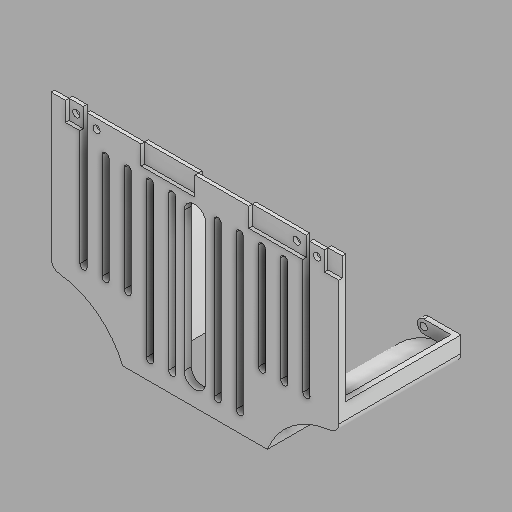
# Autodesk Inventor part: RC_CAR_TOP_PLATE
Saved by Autodesk Inventor 2025.2 (Build 292293000, 293)
## iProperties
Created: 2025-10-26
Part Number: RC_CAR_TOP_PLATE
Material: Generic
Document SubType Name: Modeling
Designer: Ben
Density: 1 g/cm^3
Appearance: Default
Author: Ben
Autodesk Inventor part; units mm, degrees
ref_plane "YZ Plane" through (0, 0, 0) normal (1, 0, 0) x (0, 1, 0)
ref_plane "XZ Plane" through (0, 0, 0) normal (0, 1, 0) x (-1, 0, 0)
ref_plane "XY Plane" through (0, 0, 0) normal (0, 0, 1) x (1, 0, 0)
sketch "Sketch1" plane through (0, 0, 0) normal (0, 0, 1) x (1, 0, 0)
  line L0 (-133.35, 0) -> (133.35, 0) projected
  line L1 (0, -231.14) -> (0, 231.14) projected
  line L2 (-44.45, -165.1) -> (44.45, 165.1) construction
  line L3 (44.45, -165.1) -> (-44.45, 165.1) construction
  line L4 (-95.25, -88.9) -> (-44.45, -88.9)
  line L5 (-44.45, 88.9) -> (-95.25, 88.9)
  line L6 (-95.25, 88.9) -> (-95.25, -88.9)
  line L7 (-95.25, -88.9) -> (-44.45, 88.9) construction
  line L8 (-44.45, -88.9) -> (-95.25, 88.9) construction
  line L9 (95.25, -88.9) -> (44.45, -88.9)
  line L10 (44.45, 88.9) -> (95.25, 88.9)
  line L11 (95.25, 88.9) -> (95.25, -88.9)
  line L12 (95.25, -88.9) -> (44.45, 88.9) construction
  line L13 (44.45, -88.9) -> (95.25, 88.9) construction
  line L14 (44.45, -165.1) -> (44.45, -88.9)
  line L15 (44.45, 88.9) -> (44.45, 165.1)
  line L16 (-44.45, 165.1) -> (-44.45, 88.9)
  line L17 (-44.45, -88.9) -> (-44.45, -165.1)
  line L18 (-31.75, 120.65) -> (31.75, 120.65)
  line L19 (31.75, 120.65) -> (31.75, 165.1)
  line L20 (-31.75, 165.1) -> (-31.75, 120.65)
  line L21 (-31.75, 120.65) -> (31.75, 165.1) construction
  line L22 (31.75, 120.65) -> (-31.75, 165.1) construction
  line L23 (-31.75, -120.65) -> (31.75, -120.65)
  line L24 (31.75, -120.65) -> (31.75, -165.1)
  line L25 (-31.75, -165.1) -> (-31.75, -120.65)
  line L26 (-31.75, -120.65) -> (31.75, -165.1) construction
  line L27 (31.75, -120.65) -> (-31.75, -165.1) construction
  line L28 (44.45, 165.1) -> (31.75, 165.1)
  line L29 (-31.75, 165.1) -> (-44.45, 165.1)
  line L30 (-44.45, -165.1) -> (-31.75, -165.1)
  line L31 (31.75, -165.1) -> (44.45, -165.1)
  point P0 (0, 0)
  point P1 (-69.85, 0)
  point P2 (69.85, 0)
  point P3 (0, 142.875)
  point P4 (0, -142.875)
  dimension "d0" = 88.9
  dimension "d1" = 330.2
  dimension "d3" = 50.8
  dimension "d4" = 12.7
  dimension "d5" = 44.45
  dimension "d27" = 76.2
  constraints: 60 end point, 12 parallel, 10 midpoint, 6 horizontal, 6 perpendicular, 4 point on line, 4 other
  measures "d0" distance of L2.end L3.end
  measures "d1" distance of L3.end L2.start
  measures "d3" distance of L4.start L4.end
  measures "d4" distance between parallel lines of L16 L20
  measures "d5" distance of L20.start L18.start
  measures "d27" distance between parallel lines of L29 L5
extrude "Extrusion1" add sketch "Sketch1" along normal blind 4.7625
sketch "Sketch3" plane through (0, 0, 4.7625) normal (0, 0, 1) x (1, 0, 0)
  line L0 (73.8188, -76.2) -> (73.8187, 76.2) construction
  line L1 (76.2, -76.2) -> (76.2, 76.2)
  line L2 (71.4375, 76.2) -> (71.4375, -76.2)
  arc A0 (71.4375, -76.2) -> (76.2, -76.2) centre (73.8188, -76.2) ccw
  arc A1 (76.2, 76.2) -> (71.4375, 76.2) centre (73.8187, 76.2) ccw
  line L3 (-73.8188, -76.2) -> (-73.8188, 76.2) construction
  line L4 (-71.4375, -76.2) -> (-71.4375, 76.2)
  line L5 (-76.2, 76.2) -> (-76.2, -76.2)
  arc A2 (-76.2, -76.2) -> (-71.4375, -76.2) centre (-73.8188, -76.2) ccw
  arc A3 (-71.4375, 76.2) -> (-76.2, 76.2) centre (-73.8188, 76.2) ccw
  line L6 (0, -231.14) -> (0, 231.14) projected
  line L7 (-133.35, 0) -> (133.35, 0) projected
  line L8 (95.25, -88.9) -> (95.25, 88.9) projected
  line L9 (59.1344, -76.2) -> (59.1344, -6.35) construction
  line L10 (61.5156, -76.2) -> (61.5156, -6.35)
  line L11 (56.7531, -6.35) -> (56.7531, -76.2)
  arc A4 (56.7531, -76.2) -> (61.5156, -76.2) centre (59.1344, -76.2) ccw
  arc A5 (61.5156, -6.35) -> (56.7531, -6.35) centre (59.1344, -6.35) ccw
  line L12 (44.45, -76.2) -> (44.45, -6.35) construction
  line L13 (44.45, -165.1) -> (44.45, -88.9) projected
  line L14 (46.8313, -76.2) -> (46.8313, -6.35)
  line L15 (42.0688, -6.35) -> (42.0688, -76.2)
  arc A6 (42.0688, -76.2) -> (46.8313, -76.2) centre (44.45, -76.2) ccw
  arc A7 (46.8313, -6.35) -> (42.0688, -6.35) centre (44.45, -6.35) ccw
  line L16 (-59.1344, -76.2) -> (-59.1344, -6.35) construction
  line L17 (-56.7531, -76.2) -> (-56.7531, -6.35)
  line L18 (-61.5156, -6.35) -> (-61.5156, -76.2)
  arc A8 (-61.5156, -76.2) -> (-56.7531, -76.2) centre (-59.1344, -76.2) ccw
  arc A9 (-56.7531, -6.35) -> (-61.5156, -6.35) centre (-59.1344, -6.35) ccw
  line L19 (-44.45, -76.2) -> (-44.45, -6.35) construction
  line L20 (-95.25, -88.9) -> (-44.45, -88.9) projected
  line L21 (-42.0687, -76.2) -> (-42.0687, -6.35)
  line L22 (-46.8313, -6.35) -> (-46.8313, -76.2)
  arc A10 (-46.8313, -76.2) -> (-42.0687, -76.2) centre (-44.45, -76.2) ccw
  arc A11 (-42.0687, -6.35) -> (-46.8313, -6.35) centre (-44.45, -6.35) ccw
  line L23 (-73.8188, -76.2) -> (-59.1344, -76.2) construction
  line L24 (-44.45, -76.2) -> (-59.1344, -76.2) construction
  line L25 (59.1344, -76.2) -> (44.45, -76.2) construction
  line L26 (73.8188, -76.2) -> (59.1344, -76.2) construction
  line L27 (29.7656, -107.95) -> (29.7656, -6.35) construction
  line L28 (44.45, 88.9) -> (44.45, 165.1) projected
  line L29 (32.1469, -107.95) -> (32.1469, -6.35)
  line L30 (27.3844, -6.35) -> (27.3844, -107.95)
  arc A12 (27.3844, -107.95) -> (32.1469, -107.95) centre (29.7656, -107.95) ccw
  arc A13 (32.1469, -6.35) -> (27.3844, -6.35) centre (29.7656, -6.35) ccw
  line L31 (-31.75, -120.65) -> (31.75, -120.65) projected
  line L32 (44.45, -76.2) -> (29.7656, -76.2) construction
  line L33 (-29.7656, -107.95) -> (-29.7656, -6.35) construction
  line L34 (-27.3844, -107.95) -> (-27.3844, -6.35)
  line L35 (-32.1469, -6.35) -> (-32.1469, -107.95)
  arc A14 (-32.1469, -107.95) -> (-27.3844, -107.95) centre (-29.7656, -107.95) ccw
  arc A15 (-27.3844, -6.35) -> (-32.1469, -6.35) centre (-29.7656, -6.35) ccw
  line L36 (-44.45, -76.2) -> (-29.7656, -76.2) construction
  line L37 (-15.0812, -107.95) -> (-15.0812, -6.35) construction
  line L38 (-12.7, -107.95) -> (-12.7, -6.35)
  line L39 (-17.4625, -6.35) -> (-17.4625, -107.95)
  arc A16 (-17.4625, -107.95) -> (-12.7, -107.95) centre (-15.0812, -107.95) ccw
  arc A17 (-12.7, -6.35) -> (-17.4625, -6.35) centre (-15.0812, -6.35) ccw
  line L40 (-29.7656, -76.2) -> (-15.0812, -76.2) construction
  line L41 (15.0812, -107.95) -> (15.0813, -6.35) construction
  line L42 (17.4625, -107.95) -> (17.4625, -6.35)
  line L43 (12.7, -6.35) -> (12.7, -107.95)
  arc A18 (12.7, -107.95) -> (17.4625, -107.95) centre (15.0812, -107.95) ccw
  arc A19 (17.4625, -6.35) -> (12.7, -6.35) centre (15.0813, -6.35) ccw
  line L44 (29.7656, -76.2) -> (15.0812, -76.2) construction
  line L45 (0, -103.1875) -> (0, -11.1125) construction
  line L46 (7.1438, -103.1875) -> (7.1438, -11.1125)
  line L47 (-7.1438, -11.1125) -> (-7.1438, -103.1875)
  arc A20 (-7.1438, -103.1875) -> (7.1438, -103.1875) centre (0, -103.1875) ccw
  arc A21 (7.1438, -11.1125) -> (-7.1438, -11.1125) centre (0, -11.1125) ccw
  line L48 (-29.7656, -110.3313) -> (29.7656, -110.3313) construction
  point P0 (0, 0)
  point P1 (73.8187, 0)
  point P2 (-73.8187, 0)
  point P3 (59.1344, -41.275)
  point P4 (44.45, -41.275)
  point P5 (-59.1344, -41.275)
  point P6 (-44.45, -41.275)
  point P7 (29.7656, -57.15)
  point P8 (-29.7656, -57.15)
  point P9 (-15.0812, -57.15)
  point P10 (15.0813, -57.15)
  point P11 (0, -57.15)
  point P12 (0, -110.3313)
  point P13 (-59.1344, -3.9687)
  point P14 (-44.45, -3.9687)
  point P15 (-29.7656, -3.9687)
  point P16 (-15.0812, -3.9687)
  point P17 (0, -3.9687)
  point P18 (15.0813, -3.9688)
  point P19 (29.7656, -3.9687)
  point P20 (44.45, -3.9688)
  point P21 (59.1344, -3.9688)
  dimension "d22" = 152.4
  dimension "d23" = 4.7625
  dimension "d24" = 19.05
  dimension "d51" = 12.7
  dimension "d53" = 14.2875
  dimension "d54" = 6.35
  constraints: 106 end point, 56 point on circle, 45 tangent, 22 centre point, 16 horizontal alignment, 14 parallel, 11 midpoint, 9 collinear, 8 equal radius, 8 perpendicular, 6 point on line, 4 vertical, 2 vertical alignment, 2 other
  measures "d22" distance of L0.end L0.start
  measures "d23" distance between parallel lines of L1 L2
  measures "d24" distance between parallel lines of L8 L1
  measures "d51" distance from line of L31 L27.start
  measures "d53" distance between parallel lines of L46 L47
  measures "d54" distance from line of L7 L12.end
extrude "Extrusion2" cut sketch "Sketch3" along normal through all both and the other way through all
fillet "Fillet1" radius 6.35 16 edges at (44.45, 165.1, 2.3813) (31.75, 165.1, 2.3813) (95.25, 88.9, 2.3813) (31.75, 120.65, 2.3813) (-31.75, 120.65, 2.3813) (-31.75, 165.1, 2.3813) (-44.45, 165.1, 2.3813) (-95.25, 88.9, 2.3813) (-95.25, -88.9, 2.3813) (-44.45, -165.1, 2.3813) (-31.75, -165.1, 2.3813) (-31.75, -120.65, 2.3813) (31.75, -120.65, 2.3813) (31.75, -165.1, 2.3813) (44.45, -165.1, 2.3813) (95.25, -88.9, 2.3813)
fillet "Fillet2" radius 50.8 4 edges at (44.45, -88.9, 2.3813) (-44.45, -88.9, 2.3813) (-44.45, 88.9, 2.3813) (44.45, 88.9, 2.3813)
sketch "Sketch4" plane through (0, 0, 4.7625) normal (0, 0, 1) x (1, 0, 0)
  line L0 (-133.35, 0) -> (133.35, 0) projected
  line L1 (0, -231.14) -> (0, 231.14) projected
  line L2 (95.25, -82.55) -> (95.25, 82.55) projected
  line L3 (95.25, 12.7) -> (-95.25, 12.7)
  line L4 (-95.25, 12.7) -> (-95.25, 165.1)
  line L5 (-95.25, 165.1) -> (95.25, 165.1)
  line L6 (95.25, 165.1) -> (95.25, 12.7)
  arc A0 (-31.75, 158.75) -> (-44.45, 158.75) centre (-38.1, 158.75) ccw projected
  point P0 (0, 0)
  point P1 (-95.25, 82.55)
  dimension "d30" = 12.7
  constraints: 8 end point, 2 parallel, 1 horizontal, 1 perpendicular, 1 point on line, 1 tangent, 1 vertical alignment
  measures "d30" distance between parallel lines of L0 L3
extrude "Extrusion3" cut sketch "Sketch4" along normal through all both and the other way through all contours L3 L4 L5 L1 | L1 L5 L6 L2 L3
sketch "Sketch5" plane through (0, 0, 4.7625) normal (0, 0, 1) x (1, 0, 0)
  line L0 (-95.25, 12.7) -> (-76.2, 12.7) projected
  line L1 (-76.2, 12.7) -> (-85.725, 12.7)
  line L2 (-85.725, 12.7) -> (-85.725, 0)
  line L3 (-85.725, 0) -> (-76.2, 0)
  line L4 (-76.2, 0) -> (-76.2, 12.7)
  line L5 (71.4375, 12.7) -> (-71.4375, 12.7) projected
  line L6 (0, 0) -> (-35.7188, 0)
  line L7 (-35.7188, 0) -> (-35.7187, 12.7)
  line L8 (-35.7187, 12.7) -> (0, 12.7)
  line L9 (0, 12.7) -> (0, 0)
  line L10 (71.4375, 12.7) -> (35.7188, 12.7)
  line L11 (35.7188, 12.7) -> (35.7188, 0)
  line L12 (35.7188, 0) -> (71.4375, 0)
  line L13 (71.4375, 0) -> (71.4375, 12.7)
  line L14 (95.25, -82.55) -> (95.25, 12.7) projected
  line L15 (95.25, 12.7) -> (85.725, 12.7)
  line L16 (85.725, 12.7) -> (85.725, 0)
  line L17 (85.725, 0) -> (95.25, 0)
  line L18 (95.25, 0) -> (95.25, 12.7)
  line L19 (95.25, 12.7) -> (76.2, 12.7) projected
  point P0 (-85.725, 12.7)
  dimension "d33" = 35.7188
  dimension "d34" = 35.7188
  constraints: 32 end point, 8 parallel, 4 horizontal, 4 perpendicular, 3 horizontal alignment, 2 midpoint, 1 coincident, 1 point on line, 1 vertical alignment
  measures "d33" distance of L6.start L6.end
  measures "d34" distance of L11.end L12.end
extrude "Extrusion4" cut sketch "Sketch5" against normal blind 2.3813
sketch "Sketch6" plane through (0, 0, 0) normal (0, 0, -1) x (-1, 0, 0)
  line L0 (95.25, 12.7) -> (95.25, -82.55) projected
  line L1 (85.725, 0) -> (95.25, 0)
  line L2 (95.25, 0) -> (95.25, 12.7)
  line L3 (95.25, 12.7) -> (85.725, 12.7)
  line L4 (85.725, 12.7) -> (85.725, 0)
  line L5 (71.4375, 12.7) -> (-71.4375, 12.7) projected
  line L6 (35.7188, 0) -> (71.4375, 0)
  line L7 (71.4375, 0) -> (71.4375, 12.7)
  line L8 (71.4375, 12.7) -> (35.7188, 12.7)
  line L9 (35.7188, 12.7) -> (35.7188, 0)
  line L10 (0, 0) -> (35.7188, 0) projected
  line L11 (0, 0) -> (-35.7188, 0)
  line L12 (-35.7188, 0) -> (-35.7188, 12.7)
  line L13 (-35.7188, 12.7) -> (0, 12.7)
  line L14 (0, 12.7) -> (0, 0)
  line L15 (-85.725, 0) -> (-85.725, 12.7) projected
  line L16 (-76.2, 12.7) -> (-76.2, -76.2) projected
  line L17 (-85.725, 0) -> (-76.2, 0)
  line L18 (-76.2, 0) -> (-76.2, 12.7)
  line L19 (-76.2, 12.7) -> (-85.725, 12.7)
  line L20 (-85.725, 12.7) -> (-85.725, 0)
  constraints: 32 end point, 8 parallel, 4 horizontal, 4 perpendicular, 1 collinear, 1 point on line
extrude "Extrusion5" cut sketch "Sketch6" against normal blind 2.3813 contours L0 L1 L4 L3 | L7 L6 L9 L5 | L14 L11 L12 L5 | L15 L19 L16 L17
sketch "Sketch7" plane through (0, 0, 0) normal (0, 0, -1) x (-1, 0, 0)
  line L0 (71.4375, 12.7) -> (71.4375, 0) projected
  line L1 (0, -231.14) -> (0, 231.14) projected
  line L2 (-35.7188, 12.7) -> (-71.4375, 12.7) projected
  line L3 (-85.725, 0) -> (-85.725, 12.7) projected
  point P0 (0, 0)
  point P1 (80.9625, 6.35)
  point P2 (65.0875, 6.35)
  point P3 (-80.9625, 6.35)
  point P4 (-65.0875, 6.35)
  dimension "d39" = 6.35
  dimension "d40" = 6.35
  dimension "d41" = 4.7625
  constraints: 3 horizontal alignment, 2 symmetric about line
  measures "d39" distance from line of L0 point (65.088, 6.35)
  measures "d40" distance from line of L2 point (-65.088, 6.35)
  measures "d41" distance from line of L3 point (-80.963, 6.35)
hole "Hole2" at (-80.9625, 6.35, 0) at (-65.0875, 6.35, 0) at (80.9625, 6.35, 0) at (65.0875, 6.35, 0) direction (0, 0, 1) diameter 4.7625 end through all
sketch "Sketch8" plane through (0, 0, 4.7625) normal (0, 0, 1) x (1, 0, 0)
  arc A0 (-44.45, -139.3461) -> (-89.6056, -88.8607) centre (-95.25, -139.3461) ccw projected
  line L0 (48.0155, -165.1) -> (-48.0155, -165.1)
  line L1 (-48.0155, -165.1) -> (-48.0155, -120.65)
  line L2 (-48.0155, -120.65) -> (48.0155, -120.65)
  line L3 (48.0155, -120.65) -> (48.0155, -165.1)
  line L4 (48.0155, -165.1) -> (-48.0155, -120.65) construction
  line L5 (-48.0155, -165.1) -> (48.0155, -120.65) construction
  arc A1 (-44.45, -158.75) -> (-31.75, -158.75) centre (-38.1, -158.75) ccw projected
  arc A2 (89.6056, -88.8607) -> (44.45, -139.3461) centre (95.25, -139.3461) ccw projected
  point P0 (0, 0)
  point P1 (0, -142.875)
  point P2 (-25.4, -120.65)
  constraints: 12 end point, 2 midpoint, 2 parallel, 2 point on circle, 1 horizontal, 1 horizontal alignment, 1 perpendicular, 1 tangent
extrude "Extrusion6" cut sketch "Sketch8" along normal through all both and the other way through all
sketch "Sketch9" plane through (0, 0, 0) normal (0, 0, -1) x (-1, 0, 0)
  arc A0 (-48.0155, -120.65) -> (-89.6056, -88.8607) centre (-95.25, -139.3461) ccw projected
  arc A1 (-95.25, -82.55) -> (-89.6056, -88.8607) centre (-88.9, -82.55) ccw projected
  arc A2 (-48.0155, -120.65) -> (-89.6056, -88.8607) centre (-95.25, -139.3461) ccw
  arc A3 (-95.25, -82.55) -> (-89.6056, -88.8607) centre (-88.9, -82.55) ccw
  arc A4 (-39.3692, -120.65) -> (-91.7772, -80.5231) centre (-95.25, -139.3461) ccw
  arc A5 (-76.2, -76.2) -> (-71.4375, -76.2) centre (-73.8188, -76.2) ccw projected
  line L0 (-95.25, -82.55) -> (-95.25, 12.7) projected
  line L1 (-91.7772, -80.5231) -> (-73.8188, -80.5231)
  line L2 (-73.8188, -71.8769) -> (-95.25, -71.8769)
  arc A6 (-73.8188, -80.5231) -> (-73.8188, -71.8769) centre (-73.8188, -76.2) ccw
  line L3 (-85.725, 12.7) -> (-95.25, 12.7) projected
  line L4 (-39.3692, -120.65) -> (-48.0155, -120.65) construction
  line L5 (-91.7772, -80.5231) -> (-91.7772, -71.8769) construction
  line L6 (48.0155, -120.65) -> (-48.0155, -120.65) construction
  circle A7 centre (-73.8188, -76.2) radius 2.3813
  line L7 (-39.3692, -120.65) -> (-48.0155, -120.65)
  line L8 (-95.25, -71.8769) -> (-95.25, -82.55)
  point P0 (0, 0)
  point P1 (-71.4375, -76.2)
  point P2 (-76.2, -76.2)
  dimension "d55" = 3.4728
  constraints: 12 end point, 8 point on circle, 5 centre point, 4 coincident, 4 tangent, 3 point on line, 2 collinear, 2 parallel, 2 perpendicular, 1 concentric
  measures "d55" distance from line of L0 L1.start
extrude "Extrusion7" add sketch "Sketch9" along normal blind 76.2
sketch "Sketch10" plane through (73.8188, -71.8769, 0) normal (0, 1, 0) x (1, 0, 0)
  line L0 (-4.3231, 0) -> (-4.3231, 76.2) projected
  line L1 (17.9585, 0) -> (17.9585, 76.2) projected
  line L2 (-4.3231, 73.025) -> (17.9585, 73.025)
  line L3 (17.9585, 73.025) -> (17.9585, 0)
  line L4 (17.9585, 0) -> (-4.3231, 0)
  line L5 (-4.3231, 0) -> (-4.3231, 73.025)
  line L6 (0, 76.2) -> (21.4313, 76.2) projected
  point P0 (-73.8188, 0)
  point P1 (17.9585, 73.025)
  dimension "d58" = 3.175
  constraints: 8 end point, 2 parallel, 1 horizontal, 1 perpendicular, 1 point on line
  measures "d58" distance between parallel lines of L6 L2
extrude "Extrusion8" cut sketch "Sketch10" against normal up to surface (8.6463 mm away)
mirror "Mirror2" about plane through (0, 0, 0) normal (1, 0, 0) of "Extrusion7", "Extrusion8"
body "Solid1"
